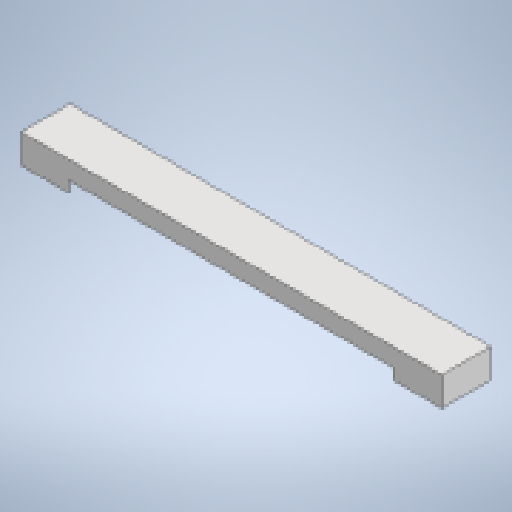
# Autodesk Inventor part: belka
Saved by Autodesk Inventor 2023 (Build 270158000, 158)
## iProperties
Created: 2025-01-12
Part Number: belka
Material: Ogólny
Document SubType Name: Modeling
Designer: kamil
Density: 1 g/cm^3
Appearance: Domyślna
Author: kamil
Autodesk Inventor part; units mm, degrees
ref_plane "YZ Plane" through (0, 0, 0) normal (1, 0, 0) x (0, 1, 0)
ref_plane "XZ Plane" through (0, 0, 0) normal (0, 1, 0) x (-1, 0, 0)
ref_plane "XY Plane" through (0, 0, 0) normal (0, 0, 1) x (1, 0, 0)
sketch "Szkic1" plane through (0, 0, 0) normal (1, 0, 0) x (0, 1, 0)
  line L0 (0, 0) -> (-3.7, 0)
  line L1 (-3.7, 0) -> (-3.7, -10)
  line L2 (-3.7, -10) -> (0, -10)
  line L3 (0, -10) -> (0, 0)
  dimension "d0" = 3.7
  dimension "d1" = 10
  constraints: 8 end point, 2 parallel, 1 horizontal, 1 perpendicular
  measures "d0" distance of L2.end L1.end
  measures "d1" distance of L1.end L0.end
extrude "Wyciągnięcie proste1" add sketch "Szkic1" along normal blind 86
sketch "Szkic2" plane through (0, -3.7, -10) normal (0, -1, 0) x (1, 0, 0)
  line L0 (0, 10) -> (0, 0) projected
  line L1 (0, 0) -> (86, 0) projected
  line L2 (86, 10) -> (86, 0) projected
  line L3 (0, 10) -> (86, 10) projected
  line L4 (0, 0) -> (10, 10)
  line L5 (0, 10) -> (86, 10) projected
  line L6 (86, 0) -> (76, 10)
  dimension "d4" = 45
  dimension "d5" = 45
  constraints: 4 end point, 2 point on line
  measures "d4" angle of L0 L4
  measures "d5" angle of L2 L6
extrude "Wyciągnięcie proste2" add sketch "Szkic2" along normal blind 2.23 contours L3 L4 L0 | L6 L3 L2
